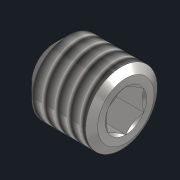
# Autodesk Inventor part: Hexagon socket set screw with flat point DIN 913 - M4x4
Saved by Autodesk Inventor 2022 (Build 260153000, 153)
## iProperties
Part Number: Hexagon socket set screw with flat point DIN 913 - M4x4
Material: 鋼、炭素鋼
Catalog Web Link: www.cadenas.de
Description: DIN 913-Hexagon socket set screw with flat point
Vendor: MISUMI
Document SubType Name: Modeling
Designer: partserver
Manufacturer: MISUMI
Mass: 0.324441 g
Surface Area: 0.768724 cm^2
Volume: 0.04133 cm^3
Density: 7.85 g/cm^3
Appearance: 半つや出し
Category: PARTsolutions
Company: MISUMI
PSOL_IDENT_0: {$CADENAS_DATA\23d-libs\misumi\metric\accessories\din_913.prj},255 {VTYP=3D},{NB=Hexagon socket set
PSOL_IDENT_1: screw with flat point DIN 913 - M4x4},{LINA=Hexagon socket set screw with flat point DIN 913 - M4x4}
PSOL_IDENT_2: ,{NN=DIN 913},{DATE=30.09.2021 08:25:08},{GEOMDATE=17.02.2014 00:00:00},{VERSION=v1},{LINEID=1000},{
PSOL_IDENT_3: WBVAR=},{WBNUMERIC=}  {NB=Gewindestift DIN 913 - M4x4},{LINA=Gewindestift DIN 913 - M4x4},{KT=X},{ID
PSOL_IDENT_4: NR=},{NENN=M4x4},{D=4.000},{D3=3.141},{P=0.700},{L=4.000},{DP=2.500},{S=2.000},{T=1.500}
NB: Headless pin DIN 913 - M4x4
NN: DIN 913
NT: Hexagon socket set screw with flat point
NBSYN: Headless pin DIN 913 - $NENN.
LINA: Headless pin DIN 913 - M4x4
CATALOG: Misumi
ROWDESC: M4x4
D: 4
D3: 3.141
P: 0.7
L: 4
DP: 2.5
S: 2
T: 1.5
SUPPLIER: MISUMI
ARTICLENO: Hexagon socket set screw with flat point DIN 913 - M4x4
BOMINFO: Hexagon socket set screw with flat point DIN 913 - M4x4
CREATOR: CADENAS GmbH
Title: Hexagon socket set screw with flat point DIN 913 - M4x4
Author: Cadenas PARTsolutions
Comments: Hexagon socket set screw with flat point
Autodesk Inventor part; units mm, degrees
sketch "Sketch_1" plane through (0, 0, 0) normal (0, 0, 1) x (1, 0, 0)
  line L0 (0.6667, 0) -> (4, 0)
  line L1 (4, 0) -> (4, -1.25)
  line L2 (4, -1.25) -> (3.25, -2)
  line L3 (3.25, -2) -> (0.248, -2)
  line L4 (0.248, -2) -> (0, -1.5705)
  line L5 (0, -1.5705) -> (0, -1.1547)
  line L6 (0, -1.1547) -> (0.6667, 0)
  line L7 (0.6667, 0) -> (4, 0)
  constraints: 16 end point
revolve "Revolution1" add sketch "Sketch_1" angle 360 about axis through (0.6667, 0, 0) along (1, 0, 0)
thread "Thread1" size "M4x0.7" class "6g" standard "ISO Metric profile" full length
sketch "Sketch_2" plane through (0, 0, 0) normal (1, 0, 0) x (0, 1, 0)
  line L0 (0, 1.1547) -> (-1, 0.5774)
  line L1 (-1, 0.5774) -> (-1, -0.5774)
  line L2 (-1, -0.5774) -> (0, -1.1547)
  line L3 (0, -1.1547) -> (1, -0.5774)
  line L4 (1, -0.5774) -> (1, 0.5774)
  line L5 (1, 0.5774) -> (0, 1.1547)
  constraints: 12 end point
extrude "Extrusion1" cut sketch "Sketch_2" along normal blind 1.5
ref_plane "IP1_XY" through (0, 0, 0) normal (1, 0, 0) x (0, 0, -1)
ref_plane "IP1_YZ" through (0, 0, 0) normal (0, 0, -1) x (0, 1, 0)
ref_plane "IP1_ZX" through (0, 0, 0) normal (0, 1, 0) x (1, 0, 0)
ref_plane "IP2_XY" through (4, 0, 0) normal (1, 0, 0) x (0, 0, -1)
ref_plane "IP2_YZ" through (4, 0, 0) normal (0, 0, -1) x (0, 1, 0)
ref_plane "IP2_ZX" through (4, 0, 0) normal (0, 1, 0) x (1, 0, 0)
body "Solid1"
